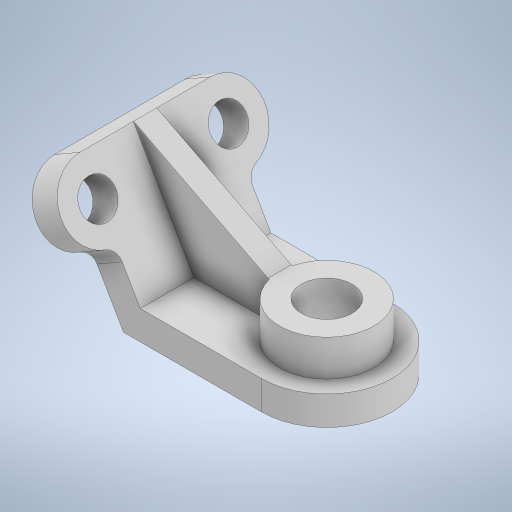
# Autodesk Inventor part: Pieza2-Tarea1
Saved by Autodesk Inventor 2024 (Build 280153000, 153)
## iProperties
Created: 2024-02-21
Part Number: Pieza2-Tarea1
Material: Genérico
Document SubType Name: Modeling
Designer: Diegolap
Mass: 492.783 g
Surface Area: 697.173 cm^2
Volume: 492.783 cm^3
Density: 1 g/cm^3
Appearance: Valor por defecto
Author: Diegolap
Autodesk Inventor part; units mm, degrees
ref_plane "YZ Plane" through (0, 0, 0) normal (1, 0, 0) x (0, 1, 0)
ref_plane "XZ Plane" through (0, 0, 0) normal (0, 1, 0) x (-1, 0, 0)
ref_plane "XY Plane" through (0, 0, 0) normal (0, 0, 1) x (1, 0, 0)
sketch "Boceto1" plane through (0, 0, 0) normal (0, 0, 1) x (1, 0, 0)
  line L0 (0, 0) -> (95, 0)
  line L1 (0, 0) -> (-47.5, 82.2724)
  line L2 (0, 0) -> (-47.5, 82.2724)
  line L3 (-47.5, 82.2724) -> (-30.1795, 92.2724)
  line L4 (-30.1795, 92.2724) -> (17.3205, 10)
  line L5 (17.3205, 10) -> (0, 0)
  line L6 (95, 0) -> (0, 0)
  line L7 (0, 0) -> (0, 20)
  line L8 (0, 20) -> (95, 20)
  line L9 (95, 20) -> (95, 0)
  point P0 (11.547, 20)
  dimension "d0" = 95
  dimension "d1" = 95
  dimension "d2" = 120
  dimension "d3" = 20
  dimension "d4" = 20
  constraints: 20 end point, 6 equal length, 2 perpendicular, 1 horizontal
  measures "d0" distance of L0.start L0.end
  measures "d1" distance of L0.start L1.end
  measures "d2" angle of L0 L1
  measures "d3" distance of L1.end L3.end
  measures "d4" distance of L8.end L0.end
extrude "Extrusión1" add sketch "Boceto1" along normal mid plane 90
sketch "Boceto2" plane through (11.547, 20, 45) normal (0, 1, 0) x (1, 0, 0)
  line L0 (83.453, 90) -> (83.453, 0) projected
  line L1 (83.453, 90) -> (83.453, 0)
  line L2 (-11.547, 0) -> (83.453, 0) projected
  arc A0 (83.453, 0) -> (83.453, 90) centre (83.453, 45) ccw
  point P0 (-11.547, 45)
  constraints: 2 end point, 2 point on circle, 1 centre point, 1 collinear, 1 tangent
extrude "Extrusión2" add sketch "Boceto2" against normal blind 20
sketch "Boceto3" plane through (11.547, 20, 45) normal (0, 1, 0) x (1, 0, 0)
  line L0 (83.453, 90) -> (-11.547, 90) projected
  line L1 (-11.547, 0) -> (83.453, 0) projected
  line L2 (83.453, 90) -> (83.453, 0)
  circle A0 centre (83.453, 45) radius 17.5
  circle A1 centre (83.453, 45) radius 32.5
  point P0 (-11.547, 45)
  dimension "d9" = 35
  dimension "d10" = 65
  constraints: 2 centre point, 2 end point, 1 coincident, 1 midpoint, 1 vertical
  measures "d9" diameter of A0
  measures "d10" diameter of A1
extrude "Extrusión3" add sketch "Boceto3" along normal blind 25 contours A1 L2 A0 | L2 A0 A1
sketch "Boceto4" plane through (0, 0, 0) normal (0, 0, 1) x (1, 0, 0)
  line L0 (-47.5, 82.2724) -> (-30.1795, 92.2724) projected
  line L1 (127.5, 45) -> (62.5, 45) projected
  line L2 (-30.1795, 92.2724) -> (62.5, 45)
  point P0 (0, 0)
  constraints: 2 end point
extrude "Nervio1" add sketch "Boceto4" along normal mid plane 16 rib yes fills toward (-38.8147, 87.2291) open curves L0 L2 L1
sketch "Boceto5" plane through (11.547, 45, 45) normal (0, 1, 0) x (1, 0, 0)
  point P0 (-11.547, 45)
sketch "Boceto6" plane through (11.547, 45, 45) normal (0, 1, 0) x (1, 0, 0)
  arc A0 (99.0174, 53) -> (67.8886, 53) centre (83.453, 45) ccw projected
  circle A1 centre (83.453, 45) radius 17.5
  point P0 (-11.547, 45)
  point P1 (67.8886, 53)
  constraints: 1 centre point, 1 coincident
extrude "Extrusión4" cut sketch "Boceto6" against normal blind 25
sketch "Boceto7" plane through (-30.1795, 92.2724, 45) normal (0.8660254, 0.5, 0) x (0, 0, -1)
  line L0 (0, 0) -> (0, -95) projected
  line L1 (0, 0) -> (0, -25)
  arc A0 (0, 0) -> (-7.1429, -48.9579) centre (0, -25) ccw
  circle A1 centre (0, -25) radius 12.5
  line L2 (0, -58.541) -> (0, -66.8712)
  arc A2 (0, -58.541) -> (-7.1429, -48.9579) centre (-10, -58.541) ccw
  point P0 (45, -95)
  point P1 (0, -50)
  point P2 (0, -37.5)
  point P3 (0, -12.5)
  dimension "d21" = 25
  dimension "d22" = 25
  dimension "d23" = 10
  constraints: 5 point on circle, 4 end point, 4 point on line, 3 centre point, 2 coincident, 2 tangent
  measures "d21" distance of L1.end L0.start
  measures "d22" diameter of A1
  measures "d23" radius of A2
extrude "Extrusión5" add sketch "Boceto7" against normal blind 20 contours L0 A1 A2 A0
sketch "Boceto8" plane through (11.547, 20, 45) normal (0.8660254, 0.5, 0) x (0, 0, -1)
  line L0 (0, 70.953) -> (0, 45.953) projected
  circle A0 centre (0, 58.453) radius 12.5
  point P0 (45, -11.547)
  constraints: 1 midpoint, 3 other
extrude "Extrusión6" cut sketch "Boceto8" against normal blind 20 contours A0 L0 picked at (3.525, 61.8151)
mirror "Simetría1" about plane through (0, 0, 0) normal (0, 0, 1) of "Extrusión5"
sketch "Boceto9" plane through (11.547, 20, -8) normal (0.8660254, 0.5, 0) x (0, 0, -1)
  line L0 (37, 70.953) -> (37, 45.953) projected
  circle A0 centre (37, 58.453) radius 12.5
  point P0 (-8, -11.547)
  point P1 (37, 45.953)
  constraints: 1 midpoint, 3 other
extrude "Extrusión7" cut sketch "Boceto9" against normal blind 20 contours L0 A0 picked at (32.2427, 55.3342)
sketch "Boceto10" plane through (95, 20, 0) normal (0, 1, 0) x (1, 0, 0)
  circle A0 centre (0, 0) radius 17.5
  point P0 (-95, 0)
  constraints: 1 centre point
extrude "Extrusión8" cut sketch "Boceto10" against normal blind 20
